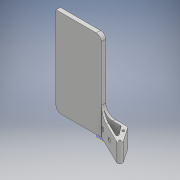
# Autodesk Inventor part: staticLink
Saved by Autodesk Inventor 2018.2 (Build 222227000, 227)
## iProperties
Created: 2017-12-31
Part Number: staticLink
Material: Generic
Document SubType Name: Modeling
Designer: mzhang
Density: 1 g/cm^3
Appearance: Default
Author: mzhang
Autodesk Inventor part; units mm, degrees
ref_plane "YZ Plane" through (0, 0, 0) normal (1, 0, 0) x (0, 1, 0)
ref_plane "XZ Plane" through (0, 0, 0) normal (0, 1, 0) x (-1, 0, 0)
ref_plane "XY Plane" through (0, 0, 0) normal (0, 0, 1) x (1, 0, 0)
ref_plane "Work Plane1" through (0, 4.778, 0) normal (0, 1, 0) x (1, 0, 0)
sketch "Sketch2" plane through (0, 4.778, 0) normal (0, 1, 0) x (1, 0, 0)
  line L0 (38.1, 0) -> (38.1, -3) projected
  line L1 (38.1, 0) -> (0, 0)
  line L2 (0, 0) -> (0, -28.4)
  line L3 (0, -28.4) -> (38.1, -28.4)
  line L4 (38.1, -28.4) -> (38.1, 0)
  circle A0 centre (28.829, -14.2) radius 1.8415
  circle A1 centre (9.271, -14.2) radius 1.8415
  point P0 (0, 0)
  point P1 (38.1, -14.2)
  point P2 (19.05, -28.4)
  point P3 (19.05, -14.2)
  dimension "d8" = 28.4
  dimension "d9" = 3.683
  dimension "d10" = 3.683
  dimension "d16" = 19.558
  constraints: 8 end point, 2 centre point, 2 midpoint, 2 parallel, 1 horizontal, 1 perpendicular
  measures "d8" distance of L2.end L1.end
  measures "d9" diameter of A0
  measures "d10" diameter of A1
  measures "d16" distance of A1.centre A0.centre
extrude "Extrusion2" add sketch "Sketch2" against normal blind 4
sketch "Sketch9" plane through (38.1, 4.778, 0) normal (0, 0, -1) x (-1, 0, 0)
  line L0 (38.1, -4) -> (0, -4) projected
  line L1 (0, -4) -> (15.0176, -4)
  circle A0 centre (-14.1784, -25.1748) radius 1.778
  circle A1 centre (-14.1784, -25.1748) radius 3.75
  line L2 (38.1, -4) -> (-12.5426, -28.5492)
  line L3 (31.3479, -4) -> (-10.5316, -24.3012)
  line L4 (-3.1089, -1.903) -> (-17.2944, -23.0884)
  line L5 (0, 0) -> (38.1, 0) projected
  arc A2 (0, 0) -> (-3.1089, -1.903) centre (0.5121, -4.3275) ccw
  line L6 (-10.5316, -24.3012) -> (4.8575, -4)
  line L7 (0, -4) -> (-0.2211, -4.3301)
  line L8 (-2.1995, -7.2849) -> (-12.092, -22.0588)
  line L9 (0, 0) -> (0, -4)
  line L10 (-13.1891, -23.6974) -> (-3.2967, -8.9235)
  circle A3 centre (-3.2967, -8.9235) radius 1.875
  line L11 (-2.1995, -7.2849) -> (-0.2211, -4.3301)
  line L12 (-2.1995, -7.2849) -> (-2.2535, -7.3655)
  line L13 (-4.3399, -10.4815) -> (-12.092, -22.0588)
  point P0 (38.1, -4.778)
  dimension "d46" = 3.556
  dimension "d47" = 7.5
  dimension "d70" = 19.558
  dimension "d71" = 3.75
  constraints: 24 end point, 8 point on circle, 3 centre point, 3 parallel, 3 point on line, 3 tangent, 2 coincident, 1 horizontal, 1 perpendicular, 3 other
  measures "d47" diameter of A1
  measures "d70" distance of A1.centre L10.end
  measures "d71" diameter of A3
extrude "Extrusion10" add sketch "Sketch9" against normal up to surface (28.4 mm away) contours L2 A1 L3 L0 | A1 | A1 L8 A3 L11 L7 L0 L6 | L4 A2 L9 L7 L11 L8 A3 A1
sketch "Sketch10" plane through (0, 0.778, 0) normal (0, -1, 0) x (1, 0, 0)
  circle A0 centre (28.829, 14.2) radius 1.8415 projected
  circle A1 centre (9.271, 14.2) radius 1.8415 projected
  circle A2 centre (28.829, 14.2) radius 3
  circle A3 centre (9.271, 14.2) radius 3
  point P0 (0, 0)
  dimension "d53" = 6
  dimension "d54" = 6
  constraints: 2 centre point, 2 coincident
  measures "d53" diameter of A2
  measures "d54" diameter of A3
extrude "Extrusion11" cut sketch "Sketch10" along normal blind 20 contours A0 | A1 | A2 | A3
fillet "Fillet5" radius 2 2 edges at (33.2425, 0.778, 14.2) (48.6316, -19.5232, 14.2)
sketch "Sketch11" plane through (0, 4.778, 28.4) normal (0, 0, 1) x (1, 0, 0)
  arc A0 (-20.0929, 0) -> (0, -0.1858) centre (-9.8968, 16.0917) ccw
  line L0 (50.6426, -28.5492) -> (0, -4) projected
  line L1 (0, -4) -> (-21.9643, -4)
  line L2 (-21.9643, -4) -> (-21.9643, 0)
  line L3 (-21.9643, 0) -> (0, 0)
  line L4 (0, 0) -> (0, -4)
  line L5 (5.3383, -6.5878) -> (-21.9643, -4)
  point P0 (0, -4.778)
  dimension "d55" = 38.1
  constraints: 10 end point, 3 point on line, 2 parallel, 2 point on circle, 1 centre point, 1 horizontal, 1 perpendicular
  measures "d55" diameter of A0
extrude "Extrusion12" add sketch "Sketch11" against normal up to surface (28.4 mm away) contours A0 L4 L1 L2 L3 | L0 L5 L1
fillet "Fillet6" radius 4 1 edges at (5.3383, -1.8098, 14.2)
sketch "Sketch12" plane through (-21.9643, 0.778, 0) normal (-0.0943581, -0.9955383, 0) x (0.9955383, -0.0943581, 0)
  line L0 (-0.3774, 28.4) -> (0, 28.4) projected
  line L1 (0, 28.4) -> (26.7035, 28.4)
  line L2 (26.7035, 28.4) -> (26.7035, 40.64)
  line L3 (26.7035, 40.64) -> (0, 40.64)
  line L4 (0, 40.64) -> (0, 28.4)
  line L5 (0, 0) -> (26.7035, 0) projected
  line L6 (21.4888, 0) -> (21.4888, 28.4) projected
  line L7 (21.4888, 28.4) -> (21.4888, 40.64)
  line L8 (-43.5998, 0) -> (26.7035, 0)
  line L9 (26.7035, 0) -> (26.7035, 111.343)
  line L10 (26.7035, 111.343) -> (-43.5998, 111.343)
  line L11 (-43.5998, 111.343) -> (-43.5998, 0)
  point P0 (21.9397, 0)
  dimension "d59" = 40.64
  constraints: 18 end point, 4 parallel, 2 horizontal, 2 perpendicular, 1 point on line, 1 vertical
  measures "d59" distance between parallel lines of L3 L5
extrude "Extrusion13" add sketch "Sketch12" along normal blind 10 starts on plane at (19.05, 4.778, 14.2) facing (0, 1, 0)
sketch "Sketch13" plane through (38.1, 4.778, 0) normal (0, 0, -1) x (-1, 0, 0)
  line L0 (33.4799, -6.5197) -> (33.8055, -9.9554) projected
  line L1 (33.4799, -6.5197) -> (112.8799, -6.5197)
  line L2 (112.8799, -6.5197) -> (112.8799, -31.9612)
  line L3 (112.8799, -31.9612) -> (33.4799, -31.9612)
  line L4 (33.4799, -31.9612) -> (33.4799, -6.5197)
  point P0 (38.1, -4.778)
  constraints: 8 end point, 2 parallel, 1 horizontal, 1 perpendicular
extrude "Extrusion14" cut sketch "Sketch13" against normal up to surface (111.343 mm away)
sketch "Sketch14" plane through (0, 4.778, 0) normal (0, 1, 0) x (1, 0, 0)
  line L0 (-72.4968, -132.6104) -> (15.2726, -132.6104)
  line L1 (15.2726, -132.6104) -> (15.2726, -93.8532)
  line L2 (15.2726, -93.8532) -> (-72.4968, -93.8532)
  line L3 (-72.4968, -93.8532) -> (-72.4968, -132.6104)
  point P0 (0, 0)
  point P1 (5.238, -111.343)
  constraints: 8 end point, 2 parallel, 1 horizontal, 1 perpendicular
extrude "Extrusion15" cut sketch "Sketch14" against normal up to surface (6.5197 mm away)
sketch "Sketch15" plane through (0, 4.778, 0) normal (0, 1, 0) x (1, 0, 0)
  line L0 (-65.9983, -137.0786) -> (5.238, -137.0786)
  line L1 (5.238, -137.0786) -> (5.238, -74.1165)
  line L2 (5.238, -74.1165) -> (-65.9983, -74.1165)
  line L3 (-65.9983, -74.1165) -> (-65.9983, -137.0786)
  line L4 (5.238, -28.4) -> (5.238, -93.8532) projected
  line L5 (-65.9983, 0) -> (-65.9983, -93.8532) projected
  point P0 (0, 0)
  dimension "d74" = 0
  dimension "d75" = 0
  constraints: 8 end point, 2 parallel, 1 horizontal, 1 perpendicular
  measures "d74" distance between parallel lines of L4 L1
  measures "d75" distance between parallel lines of L5 L3
extrude "Extrusion16" add sketch "Sketch15" against normal up to surface (6.5197 mm away)
fillet "Fillet7" radius 15 1 edges at (4.9291, 1.5182, 28.4)
sketch "Sketch16" plane through (5.238, -1.7417, 74.1165) normal (0, 0, -1) x (-1, 0, 0)
  line L0 (0, 6.5197) -> (0.6179, 0) projected
  line L1 (0, 6.5197) -> (0, 0) projected
  line L2 (0.6179, 0) -> (0, 0) projected
  line L3 (71.2363, 0) -> (70.6184, 6.5197) projected
  line L4 (71.2363, 6.5197) -> (71.2363, 0) projected
  line L5 (70.6184, 6.5197) -> (71.2363, 6.5197) projected
  point P0 (5.238, 1.7417)
extrude "Extrusion17" cut sketch "Sketch16" against normal up to surface (62.9621 mm away)
fillet "Fillet10" radius 8 2 edges at (4.9291, 1.5182, 137.0786) (-65.6893, 1.5182, 0)
body "Solid1"
